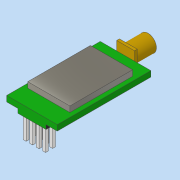
# Autodesk Inventor part: SPIRadio
Saved by Autodesk Inventor 2017.3 (Build 213256000, 256)
## iProperties
Created: 2018-07-15
Part Number: SPIRadio
Material: ABS Plastic
Document SubType Name: Modeling
Designer: Derek Wider
Density: 1.06 g/cm^3
Appearance: Smooth - White
Author: Derek Wider
Autodesk Inventor part; units mm, degrees
ref_plane "YZ Plane" through (0, 0, 0) normal (1, 0, 0) x (0, 1, 0)
ref_plane "XZ Plane" through (0, 0, 0) normal (0, 1, 0) x (-1, 0, 0)
ref_plane "XY Plane" through (0, 0, 0) normal (0, 0, 1) x (1, 0, 0)
sketch "Sketch1" plane through (0, 0, 0) normal (0, 1, 0) x (-1, 0, 0)
  line L0 (0, 0) -> (18, 0)
  line L1 (18, 0) -> (18, -33.3)
  line L2 (18, -33.3) -> (0, -33.3)
  line L3 (0, -33.3) -> (0, 0)
  dimension "d0" = 33.3
  dimension "d1" = 18
  constraints: 8 end point, 2 parallel, 1 horizontal, 1 perpendicular
  measures "d0" distance of L2.end L0.start
  measures "d1" distance of L0.start L0.end
extrude "Extrusion1" add sketch "Sketch1" along normal blind 2
sketch "Sketch2" plane through (0, 2, 0) normal (0, 1, 0) x (1, 0, 0)
  line L0 (-16.5, 6) -> (-1.5, 6)
  line L1 (-1.5, 6) -> (-1.5, 28.3)
  line L2 (-1.5, 28.3) -> (-16.5, 28.3)
  line L3 (-16.5, 28.3) -> (-16.5, 6)
  line L4 (-18, 0) -> (0, 0) projected
  line L5 (0, 33.3) -> (-18, 33.3) projected
  line L6 (-18, 33.3) -> (-18, 0) projected
  line L7 (0, 0) -> (0, 33.3) projected
  dimension "d4" = 6
  dimension "d5" = 5
  dimension "d6" = 1.5
  dimension "d7" = 1.5
  constraints: 8 end point, 2 parallel, 1 horizontal, 1 perpendicular
  measures "d4" distance between parallel lines of L4 L0
  measures "d5" distance between parallel lines of L5 L2
  measures "d6" distance between parallel lines of L6 L3
  measures "d7" distance between parallel lines of L7 L1
extrude "Extrusion2" add sketch "Sketch2" along normal blind 2 contours L3 L2 L1 L0
sketch "Sketch3" plane through (0, 0, -33.3) normal (0, 0, -1) x (-1, 0, 0)
  line L0 (18, 0) -> (0, 0) construction
  line L1 (18, 0) -> (18, 2) construction
  line L2 (0, 2) -> (18, 2) construction
  line L3 (0, 0) -> (0, 2) construction
  line L4 (5.825, 5.2) -> (12.175, 5.2)
  line L5 (12.175, 5.2) -> (12.175, -1.15)
  line L6 (12.175, -1.15) -> (5.825, -1.15)
  line L7 (5.825, -1.15) -> (5.825, 5.2)
  point P0 (0, 0)
  point P1 (9, 5.2)
  point P2 (9, 2)
  dimension "d10" = 6.35
  dimension "d11" = 6.35
  dimension "d12" = 3.2
  constraints: 8 end point, 2 midpoint, 2 parallel, 1 horizontal, 1 perpendicular, 1 vertical alignment
  measures "d10" distance of L6.end L4.start
  measures "d11" distance of L4.start L4.end
  measures "d12" distance between parallel lines of L4 L2
extrude "Extrusion3" add sketch "Sketch3" along normal blind 1
sketch "Sketch4" plane through (0, 0, -34.3) normal (0, 0, -1) x (-1, 0, 0)
  line L0 (12.175, 5.2) -> (5.825, 5.2) construction
  line L1 (5.825, 5.2) -> (5.825, -1.15) construction
  line L2 (5.825, -1.15) -> (12.175, -1.15) construction
  line L3 (12.175, -1.15) -> (12.175, 5.2) construction
  circle A0 centre (9, 2.025) radius 3
  point P0 (0, 0)
  dimension "d15" = 6
  constraints: 1 centre point
  measures "d15" diameter of A0
extrude "Extrusion4" add sketch "Sketch4" along normal blind 7
sketch "Sketch5" plane through (0, 0, 0) normal (0, -1, 0) x (1, 0, 0)
  line L0 (-18, 0) -> (0, 0) projected
  line L1 (-4, 0) -> (-14, 0)
  line L2 (-14, 0) -> (-14, -5)
  line L3 (-14, -5) -> (-4, -5)
  line L4 (-4, -5) -> (-4, 0)
  point P0 (-9, -5)
  point P1 (-9, 0)
  dimension "d18" = 5
  dimension "d19" = 10
  constraints: 8 end point, 2 midpoint, 2 parallel, 1 horizontal, 1 perpendicular, 1 point on line, 1 vertical alignment
  measures "d18" distance of L3.end L1.start
  measures "d19" distance of L2.end L3.end
extrude "Extrusion5" add sketch "Sketch5" along normal blind 1.5
sketch "Sketch6" plane through (0, -1.5, 0) normal (0, -1, 0) x (1, 0, 0)
  line L0 (-6, -1.8409) -> (-5, -1.8409)
  line L1 (-5, -1.8409) -> (-5, -0.8409)
  line L2 (-5, -0.8409) -> (-6, -0.8409)
  line L3 (-6, -0.8409) -> (-6, -1.8409)
  line L4 (-6, -4.3409) -> (-5, -4.3409)
  line L5 (-5, -4.3409) -> (-5, -3.3409)
  line L6 (-5, -3.3409) -> (-6, -3.3409)
  line L7 (-6, -3.3409) -> (-6, -4.3409)
  line L8 (-4, -5) -> (-4, 0) projected
  point P0 (0, 0)
  dimension "d22" = 1
  dimension "d23" = 1
  dimension "d24" = 1
  dimension "d25" = 1.5
  dimension "d26" = 1
  constraints: 16 end point, 4 parallel, 2 horizontal, 2 perpendicular, 1 vertical alignment
  measures "d22" distance of L1.end L2.end
  measures "d23" distance of L0.end L1.end
  measures "d24" distance of L4.end L5.end
  measures "d25" distance between parallel lines of L6 L0
  measures "d26" distance between parallel lines of L1 L8
extrude "Extrusion6" add sketch "Sketch6" along normal blind 8
pattern_linear "Rectangular Pattern1" count 4 spacing 2.3 along (-1, 0, 0) of "Extrusion6"
body "Solid1"
